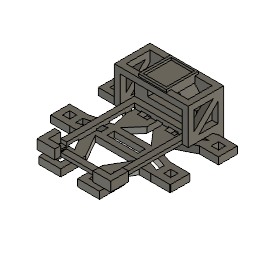
Proto-Board housing (Autodesk Fusion 360 design; units mm, degrees)
Autodesk Fusion 360 part; units mm, degrees
(part 1 of 2)
sketch "Sketch1" plane through (0, 0, 0) normal (0, 0, 1) x (1, 0, 0)
  line L0 (0, 0) -> (7, 0) construction
  line L1 (7, 0) -> (7, -7) construction
  line L2 (7, -7) -> (0, -7) construction
  line L3 (0, -7) -> (0, 0) construction
  line L4 (7, -3.5) -> (23, -3.5) construction
  line L5 (23, 0) -> (30, 0) construction
  line L6 (30, 0) -> (30, -7) construction
  line L7 (30, -7) -> (23, -7) construction
  line L8 (23, -7) -> (23, 0) construction
  line L9 (0, 0) -> (-25, 0) construction
  line L10 (30, 0) -> (55, 0) construction
  line L11 (-25, 0) -> (-30, 0) construction
  line L12 (-30, 0) -> (-30, 5) construction
  line L13 (-30, 5) -> (-25, 5) construction
  line L14 (-25, 5) -> (-25, 0) construction
  line L15 (55, 0) -> (60, 0) construction
  line L16 (60, 0) -> (60, 5) construction
  line L17 (60, 5) -> (55, 5) construction
  line L18 (55, 5) -> (55, 0) construction
  line L19 (-25, 0) -> (-25, -35) construction
  line L20 (-30, -35) -> (-25, -35) construction
  line L21 (-25, -35) -> (-25, -40) construction
  line L22 (-25, -40) -> (-30, -40) construction
  line L23 (-30, -40) -> (-30, -35) construction
  line L24 (55, 0) -> (55, -35) construction
  line L25 (55, -35) -> (60, -35) construction
  line L26 (60, -35) -> (60, -40) construction
  line L27 (60, -40) -> (55, -40) construction
  line L28 (55, -40) -> (55, -35) construction
  line L29 (15, -3.5) -> (15, -30) construction
  line L30 (15, -30) -> (2.5, -30) construction
  line L31 (2.5, -30) -> (27.5, -30) construction
  line L32 (27.5, -30) -> (27.5, -35) construction
  line L33 (27.5, -35) -> (2.5, -35) construction
  line L34 (2.5, -35) -> (2.5, -30) construction
  line L35 (2.5, -35) -> (2.5, -65) construction
  line L36 (27.5, -35) -> (27.5, -65) construction
  line L37 (2.5, -65) -> (-5, -65) construction
  line L38 (-5, -65) -> (-5, -75) construction
  line L39 (-5, -75) -> (2.5, -75) construction
  line L40 (2.5, -75) -> (2.5, -65) construction
  line L41 (27.5, -65) -> (35, -65) construction
  line L42 (35, -65) -> (35, -75) construction
  line L43 (35, -75) -> (27.5, -75) construction
  line L44 (27.5, -75) -> (27.5, -65) construction
  line L45 (-5, -65) -> (-5.5, -65) construction
  line L46 (-5.5, -65) -> (-5.5, -64.5) construction
  line L47 (-5.5, -64.5) -> (-5, -64.5) construction
  line L48 (-5, -64.5) -> (-5, -65) construction
  line L49 (-5.5, -64.5) -> (3, -64.5)
  line L50 (3, -64.5) -> (3, -75.5)
  line L51 (3, -75.5) -> (-5.5, -75.5)
  line L52 (-5.5, -75.5) -> (-5.5, -64.5)
  line L53 (27.5, -65) -> (27, -65) construction
  line L54 (27, -65) -> (27, -64.5) construction
  line L55 (27, -64.5) -> (27.5, -64.5) construction
  line L56 (27.5, -64.5) -> (27.5, -65) construction
  line L57 (27, -64.5) -> (35.5, -64.5)
  line L58 (35.5, -64.5) -> (35.5, -75.5)
  line L59 (35.5, -75.5) -> (27, -75.5)
  line L60 (27, -75.5) -> (27, -64.5)
  line L61 (2.5, -30) -> (2, -30) construction
  line L62 (2, -30) -> (2, -29.5) construction
  line L63 (2, -29.5) -> (2.5, -29.5) construction
  line L64 (2.5, -29.5) -> (2.5, -30) construction
  line L65 (-30, -35) -> (-30.5, -35) construction
  line L66 (-30.5, -35) -> (-30.5, -34.5) construction
  line L67 (-30.5, -34.5) -> (-30, -34.5) construction
  line L68 (-30, -34.5) -> (-30, -35) construction
  line L69 (-30.5, -34.5) -> (-24.5, -34.5)
  line L70 (-24.5, -34.5) -> (-24.5, -40.5)
  line L71 (-24.5, -40.5) -> (-30.5, -40.5)
  line L72 (-30.5, -40.5) -> (-30.5, -34.5)
  line L73 (-30, 5) -> (-30.5, 5) construction
  line L74 (-30.5, 5) -> (-30.5, 5.5) construction
  line L75 (-30.5, 5.5) -> (-30, 5.5) construction
  line L76 (-30, 5.5) -> (-30, 5) construction
  line L77 (-30.5, 5.5) -> (-24.5, 5.5)
  line L78 (-24.5, 5.5) -> (-24.5, -0.5)
  line L79 (-24.5, -0.5) -> (-30.5, -0.5)
  line L80 (-30.5, -0.5) -> (-30.5, 5.5)
  line L81 (0, 0) -> (-0.5, 0) construction
  line L82 (-0.5, 0) -> (-0.5, 0.5) construction
  line L83 (-0.5, 0.5) -> (0, 0.5) construction
  line L84 (0, 0.5) -> (0, 0) construction
  line L85 (-0.5, 0.5) -> (7.5, 0.5)
  line L86 (7.5, 0.5) -> (7.5, -7.5)
  line L87 (7.5, -7.5) -> (-0.5, -7.5)
  line L88 (-0.5, -7.5) -> (-0.5, 0.5)
  line L89 (23, 0) -> (22.5, 0) construction
  line L90 (22.5, 0) -> (22.5, 0.5) construction
  line L91 (22.5, 0.5) -> (23, 0.5) construction
  line L92 (23, 0.5) -> (23, 0) construction
  line L93 (22.5, 0.5) -> (30.5, 0.5)
  line L94 (30.5, 0.5) -> (30.5, -7.5)
  line L95 (30.5, -7.5) -> (22.5, -7.5)
  line L96 (22.5, -7.5) -> (22.5, 0.5)
  line L97 (55, 5) -> (54.5, 5) construction
  line L98 (54.5, 5) -> (54.5, 5.5) construction
  line L99 (54.5, 5.5) -> (55, 5.5) construction
  line L100 (55, 5.5) -> (55, 5) construction
  line L101 (54.5, 5.5) -> (60.5, 5.5)
  line L102 (60.5, 5.5) -> (60.5, -0.5)
  line L103 (60.5, -0.5) -> (54.5, -0.5)
  line L104 (54.5, -0.5) -> (54.5, 5.5)
  line L105 (54.5, -34.5) -> (60.5, -34.5)
  line L106 (60.5, -34.5) -> (60.5, -40.5)
  line L107 (60.5, -40.5) -> (54.5, -40.5)
  line L108 (54.5, -40.5) -> (54.5, -34.5)
  line L109 (60.5, -40.5) -> (65.5, -40.5) construction
  line L110 (65.5, -40.5) -> (65.5, -45.5) construction
  line L111 (65.5, -45.5) -> (60.5, -45.5) construction
  line L112 (60.5, -45.5) -> (60.5, -40.5) construction
  line L113 (35.5, -75.5) -> (40.5, -75.5) construction
  line L114 (40.5, -75.5) -> (40.5, -80.5) construction
  line L115 (40.5, -80.5) -> (35.5, -80.5) construction
  line L116 (35.5, -80.5) -> (35.5, -75.5) construction
  line L117 (40.5, -80.5) -> (65.5, -45.5)
  line L118 (60.5, -0.5) -> (65.5, -0.5) construction
  line L119 (65.5, -0.5) -> (65.5, -45.5)
  line L120 (-5.5, -75.5) -> (-10.5, -75.5) construction
  line L121 (-10.5, -75.5) -> (-10.5, -80.5) construction
  line L122 (-10.5, -80.5) -> (-5.5, -80.5) construction
  line L123 (-5.5, -80.5) -> (-5.5, -75.5) construction
  line L124 (-10.5, -80.5) -> (40.5, -80.5)
  line L125 (-30.5, -40.5) -> (-35.5, -40.5) construction
  line L126 (-35.5, -40.5) -> (-35.5, -45.5) construction
  line L127 (-35.5, -45.5) -> (-30.5, -45.5) construction
  line L128 (-30.5, -45.5) -> (-30.5, -40.5) construction
  line L129 (-35.5, -45.5) -> (-10.5, -80.5)
  line L130 (2, -29.5) -> (28, -29.5)
  line L131 (28, -29.5) -> (28, -35.5)
  line L132 (28, -35.5) -> (2, -35.5)
  line L133 (2, -35.5) -> (2, -29.5)
  line L134 (-30.5, -0.5) -> (-35.5, -0.5) construction
  line L135 (-35.5, -45.5) -> (-35.5, -0.5)
  line L136 (-30.5, 5.5) -> (-35.5, 5.5) construction
  line L137 (-35.5, 5.5) -> (-35.5, 10.5) construction
  line L138 (-35.5, 10.5) -> (-30.5, 10.5) construction
  line L139 (-30.5, 10.5) -> (-30.5, 5.5) construction
  line L140 (-35.5, -0.5) -> (-35.5, 10.5)
  line L141 (-24.5, 5.5) -> (-19.5, 5.5) construction
  line L142 (-19.5, 5.5) -> (-19.5, 10.5) construction
  line L143 (-19.5, 10.5) -> (-24.5, 10.5) construction
  line L144 (-24.5, 10.5) -> (-24.5, 5.5) construction
  line L145 (-35.5, 10.5) -> (-19.5, 10.5)
  line L146 (-0.5, 0.5) -> (-5.5, 0.5) construction
  line L147 (-5.5, 0.5) -> (-5.5, 5.5) construction
  line L148 (-5.5, 5.5) -> (-0.5, 5.5) construction
  line L149 (-0.5, 5.5) -> (-0.5, 0.5) construction
  line L150 (-19.5, 10.5) -> (-5.5, 5.5)
  line L151 (7.5, 0.5) -> (12.5, 0.5) construction
  line L152 (12.5, 0.5) -> (12.5, 5.5) construction
  line L153 (12.5, 5.5) -> (7.5, 5.5) construction
  line L154 (7.5, 5.5) -> (7.5, 0.5) construction
  line L155 (-5.5, 5.5) -> (12.5, 5.5)
  line L156 (30.5, 0.5) -> (35.5, 0.5) construction
  line L157 (35.5, 0.5) -> (35.5, 5.5) construction
  line L158 (35.5, 5.5) -> (30.5, 5.5) construction
  line L159 (30.5, 5.5) -> (30.5, 0.5) construction
  line L160 (12.5, 5.5) -> (35.5, 5.5)
  line L161 (54.5, 5.5) -> (49.5, 5.5) construction
  line L162 (49.5, 5.5) -> (49.5, 10.5) construction
  line L163 (49.5, 10.5) -> (54.5, 10.5) construction
  line L164 (54.5, 10.5) -> (54.5, 5.5) construction
  line L165 (35.5, 5.5) -> (49.5, 10.5)
  line L166 (60.5, 5.5) -> (65.5, 5.5) construction
  line L167 (65.5, 5.5) -> (65.5, 10.5) construction
  line L168 (65.5, 10.5) -> (60.5, 10.5) construction
  line L169 (60.5, 10.5) -> (60.5, 5.5) construction
  line L170 (49.5, 10.5) -> (65.5, 10.5)
  line L171 (65.5, 10.5) -> (65.5, -0.5)
  line L172 (30.5, -7.5) -> (35.5, -7.5) construction
  line L173 (35.5, -7.5) -> (35.5, -12.5) construction
  line L174 (35.5, -12.5) -> (30.5, -12.5) construction
  line L175 (30.5, -12.5) -> (30.5, -7.5) construction
  line L176 (54.5, -0.5) -> (49.5, -0.5) construction
  line L177 (49.5, -0.5) -> (49.5, -5.5) construction
  line L178 (49.5, -5.5) -> (54.5, -5.5) construction
  line L179 (54.5, -5.5) -> (54.5, -0.5) construction
  line L180 (54.5, -34.5) -> (49.5, -34.5) construction
  line L181 (49.5, -34.5) -> (49.5, -29.5) construction
  line L182 (49.5, -29.5) -> (54.5, -29.5) construction
  line L183 (54.5, -29.5) -> (54.5, -34.5) construction
  line L184 (28, -29.5) -> (33, -29.5) construction
  line L185 (33, -29.5) -> (33, -24.5) construction
  line L186 (33, -24.5) -> (28, -24.5) construction
  line L187 (28, -24.5) -> (28, -29.5) construction
  line L188 (33, -24.5) -> (35.5, -12.5)
  line L189 (35.5, -12.5) -> (49.5, -5.5)
  line L190 (49.5, -5.5) -> (49.5, -29.5)
  line L191 (33, -24.5) -> (49.5, -29.5)
  line L192 (7.5, -7.5) -> (12.5, -7.5) construction
  line L193 (12.5, -7.5) -> (12.5, -12.5) construction
  line L194 (12.5, -12.5) -> (7.5, -12.5) construction
  line L195 (7.5, -12.5) -> (7.5, -7.5) construction
  line L196 (22.5, -7.5) -> (17.5, -7.5) construction
  line L197 (17.5, -7.5) -> (17.5, -12.5) construction
  line L198 (17.5, -12.5) -> (22.5, -12.5) construction
  line L199 (22.5, -12.5) -> (22.5, -7.5) construction
  line L200 (-0.5, -7.5) -> (-5.5, -7.5) construction
  line L201 (-5.5, -7.5) -> (-5.5, -12.5) construction
  line L202 (-5.5, -12.5) -> (-0.5, -12.5) construction
  line L203 (-0.5, -12.5) -> (-0.5, -7.5) construction
  line L204 (2, -29.5) -> (-3, -29.5) construction
  line L205 (-3, -29.5) -> (-3, -24.5) construction
  line L206 (-3, -24.5) -> (2, -24.5) construction
  line L207 (2, -24.5) -> (2, -29.5) construction
  line L208 (-24.5, -0.5) -> (-19.5, -0.5) construction
  line L209 (-19.5, -0.5) -> (-19.5, -5.5) construction
  line L210 (-19.5, -5.5) -> (-24.5, -5.5) construction
  line L211 (-24.5, -5.5) -> (-24.5, -0.5) construction
  line L212 (-24.5, -34.5) -> (-19.5, -34.5) construction
  line L213 (-19.5, -34.5) -> (-19.5, -29.5) construction
  line L214 (-19.5, -29.5) -> (-24.5, -29.5) construction
  line L215 (-24.5, -29.5) -> (-24.5, -34.5) construction
  line L216 (-19.5, -5.5) -> (-19.5, -29.5)
  line L217 (-19.5, -29.5) -> (-3, -24.5)
  line L218 (-3, -24.5) -> (-5.5, -12.5)
  line L219 (-5.5, -12.5) -> (-19.5, -5.5)
  line L220 (3, -64.5) -> (8, -64.5) construction
  line L221 (8, -64.5) -> (8, -59.5) construction
  line L222 (8, -59.5) -> (3, -59.5) construction
  line L223 (3, -59.5) -> (3, -64.5) construction
  line L224 (27, -64.5) -> (22, -64.5) construction
  line L225 (22, -64.5) -> (22, -59.5) construction
  line L226 (22, -59.5) -> (27, -59.5) construction
  line L227 (27, -59.5) -> (27, -64.5) construction
  line L228 (2, -35.5) -> (-3, -35.5) construction
  line L229 (-3, -35.5) -> (-3, -40.5) construction
  line L230 (-3, -40.5) -> (2, -40.5) construction
  line L231 (2, -40.5) -> (2, -35.5) construction
  line L232 (28, -35.5) -> (33, -35.5) construction
  line L233 (33, -35.5) -> (33, -40.5) construction
  line L234 (33, -40.5) -> (28, -40.5) construction
  line L235 (28, -40.5) -> (28, -35.5) construction
  line L236 (-3, -40.5) -> (8, -59.5)
  line L237 (8, -59.5) -> (22, -59.5)
  line L238 (22, -59.5) -> (33, -40.5)
  line L239 (33, -40.5) -> (-3, -40.5)
  dimension "d1" = 7
  dimension "d2" = 7
  dimension "d3" = 16
  dimension "d4" = 25
  dimension "d5" = 25
  dimension "d6" = 26.5
  dimension "d7" = 12.5
  dimension "d8" = 25
  dimension "d9" = 5
  dimension "d10" = 30
  dimension "d11" = 7.5
  dimension "d12" = 10
  dimension "d13" = 7.5
  dimension "d14" = 10
  dimension "d15" = 0.5
  dimension "d16" = 0.5
  dimension "d17" = 8.5
  dimension "d18" = 11
  dimension "d19" = 0.5
  dimension "d20" = 0.5
  dimension "d21" = 8.5
  dimension "d22" = 11
  dimension "d23" = 0.5
  dimension "d24" = 0.5
  dimension "d27" = 5
  dimension "d28" = 5
  dimension "d29" = 5
  dimension "d30" = 5
  dimension "d31" = 5
  dimension "d32" = 5
  dimension "d33" = 5
  dimension "d34" = 5
  dimension "d35" = 5
  dimension "d36" = 26
  dimension "d37" = 6
  dimension "d38" = 5
  dimension "d39" = 5
  dimension "d40" = 5
  dimension "d41" = 5
  dimension "d42" = 5
  dimension "d43" = 5
  dimension "d44" = 5
  dimension "d45" = 5
  dimension "d46" = 5
  dimension "d47" = 5
  dimension "d48" = 5
  dimension "d49" = 5
  dimension "d50" = 5
  dimension "d51" = 5
  dimension "d52" = 5
  dimension "d53" = 5
  dimension "d54" = 5
  dimension "d55" = 5
  dimension "d56" = 5
  dimension "d57" = 5
  dimension "d58" = 5
  dimension "d59" = 5
  dimension "d60" = 5
  dimension "d61" = 5
  dimension "d62" = 5
  dimension "d63" = 5
  dimension "d64" = 5
  dimension "d65" = 5
  dimension "d66" = 5
  dimension "d67" = 5
  dimension "d68" = 5
  dimension "d69" = 5
  dimension "d70" = 5
  dimension "d71" = 5
  dimension "d72" = 5
  dimension "d73" = 5
  dimension "d74" = 5
  dimension "d75" = 5
  dimension "d76" = 5
  dimension "d77" = 5
  dimension "d78" = 5
  dimension "d79" = 5
  dimension "d80" = 5
  constraint horizontal L0
  constraint vertical L1
  constraint horizontal L2
  constraint vertical L3
  constraint coincident L0.start L3.end
  constraint midpoint L1 L4.start
  constraint perpendicular L1 L4
  constraint horizontal L5
  constraint vertical L6
  constraint horizontal L7
  constraint vertical L8
  constraint perpendicular L3 L9
  constraint perpendicular L6 L10
  constraint horizontal L11
  constraint vertical L12
  constraint horizontal L13
  constraint vertical L14
  constraint horizontal L15
  constraint vertical L16
  constraint horizontal L17
  constraint vertical L18
  constraint perpendicular L11 L19
  constraint horizontal L20
  constraint vertical L21
  constraint horizontal L22
  constraint vertical L23
  constraint perpendicular L10 L24
  constraint horizontal L25
  constraint vertical L26
  constraint horizontal L27
  constraint vertical L28
  constraint midpoint L4 L29.start
  constraint perpendicular L4 L29
  constraint perpendicular L29 L30
  constraint horizontal L31
  constraint vertical L32
  constraint horizontal L33
  constraint vertical L34
  constraint perpendicular L33 L35
  constraint perpendicular L33 L36
  constraint horizontal L37
  constraint vertical L38
  constraint horizontal L39
  constraint vertical L40
  constraint horizontal L41
  constraint vertical L42
  constraint horizontal L43
  constraint vertical L44
  constraint horizontal L45
  constraint vertical L46
  constraint horizontal L47
  constraint vertical L48
  constraint horizontal L49
  constraint vertical L50
  constraint horizontal L51
  constraint vertical L52
  constraint horizontal L53
  constraint vertical L54
  constraint horizontal L55
  constraint vertical L56
  constraint horizontal L57
  constraint vertical L58
  constraint horizontal L59
  constraint vertical L60
  constraint horizontal L61
  constraint vertical L62
  constraint horizontal L63
  constraint vertical L64
  constraint horizontal L65
  constraint vertical L66
  constraint horizontal L67
  constraint vertical L68
  constraint horizontal L69
  constraint vertical L70
  constraint horizontal L71
  constraint vertical L72
  constraint horizontal L73
  constraint vertical L74
  constraint horizontal L75
  constraint vertical L76
  constraint horizontal L77
  constraint vertical L78
  constraint horizontal L79
  constraint vertical L80
  constraint horizontal L81
  constraint vertical L82
  constraint horizontal L83
  constraint vertical L84
  constraint horizontal L85
  constraint vertical L86
  constraint horizontal L87
  constraint vertical L88
  constraint horizontal L89
  constraint vertical L90
  constraint horizontal L91
  constraint vertical L92
  constraint horizontal L93
  constraint vertical L94
  constraint horizontal L95
  constraint vertical L96
  constraint horizontal L97
  constraint vertical L98
  constraint horizontal L99
  constraint vertical L100
  constraint horizontal L101
  constraint vertical L102
  constraint horizontal L103
  constraint vertical L104
  constraint horizontal L105
  constraint vertical L106
  constraint horizontal L107
  constraint vertical L108
  constraint horizontal L109
  constraint vertical L110
  constraint horizontal L111
  constraint vertical L112
  constraint horizontal L113
  constraint vertical L114
  constraint horizontal L115
  constraint vertical L116
  constraint perpendicular L102 L118
  constraint perpendicular L111 L119
  constraint horizontal L120
  constraint vertical L121
  constraint horizontal L122
  constraint vertical L123
  constraint horizontal L125
  constraint vertical L126
  constraint horizontal L127
  constraint vertical L128
  constraint horizontal L130
  constraint vertical L131
  constraint horizontal L132
  constraint vertical L133
  constraint perpendicular L80 L134
  constraint perpendicular L134 L135
  constraint horizontal L136
  constraint vertical L137
  constraint horizontal L138
  constraint vertical L139
  constraint horizontal L141
  constraint vertical L142
  constraint horizontal L143
  constraint vertical L144
  constraint horizontal L146
  constraint vertical L147
  constraint horizontal L148
  constraint vertical L149
  constraint horizontal L151
  constraint vertical L152
  constraint horizontal L153
  constraint vertical L154
  constraint horizontal L156
  constraint vertical L157
  constraint horizontal L158
  constraint vertical L159
  constraint perpendicular L157 L160
  constraint horizontal L161
  constraint vertical L162
  constraint horizontal L163
  constraint vertical L164
  constraint horizontal L166
  constraint vertical L167
  constraint horizontal L168
  constraint vertical L169
  constraint horizontal L172
  constraint vertical L173
  constraint horizontal L174
  constraint vertical L175
  constraint horizontal L176
  constraint vertical L177
  constraint horizontal L178
  constraint vertical L179
  constraint horizontal L180
  constraint vertical L181
  constraint horizontal L182
  constraint vertical L183
  constraint horizontal L184
  constraint vertical L185
  constraint horizontal L186
  constraint vertical L187
  constraint perpendicular L182 L190
  constraint horizontal L192
  constraint vertical L193
  constraint horizontal L194
  constraint vertical L195
  constraint horizontal L196
  constraint vertical L197
  constraint horizontal L198
  constraint vertical L199
  constraint horizontal L200
  constraint vertical L201
  constraint horizontal L202
  constraint vertical L203
  constraint horizontal L204
  constraint vertical L205
  constraint horizontal L206
  constraint vertical L207
  constraint horizontal L208
  constraint vertical L209
  constraint horizontal L210
  constraint vertical L211
  constraint horizontal L212
  constraint vertical L213
  constraint horizontal L214
  constraint vertical L215
  constraint perpendicular L214 L216
  constraint horizontal L220
  constraint vertical L221
  constraint horizontal L222
  constraint vertical L223
  constraint horizontal L224
  constraint vertical L225
  constraint horizontal L226
  constraint vertical L227
  constraint horizontal L228
  constraint vertical L229
  constraint horizontal L230
  constraint vertical L231
  constraint horizontal L232
  constraint vertical L233
  constraint horizontal L234
  constraint vertical L235
  measures "d1" distance of L0.start L0.end
  measures "d2" distance of L0.start L2.end
  measures "d3" distance of L4.start L4.end
  measures "d4" distance of L0.start L9.end
  measures "d5" distance of L5.end L10.end
  measures "d6" distance of L29.start L29.end
  measures "d7" distance of L29.end L30.end
  measures "d8" distance of L30.end L31.end
  measures "d9" distance of L30.end L33.end
  measures "d10" distance of L33.end L35.end
  measures "d11" distance of L35.end L37.end
  measures "d12" distance of L35.end L39.end
  measures "d13" distance of L36.end L41.end
  measures "d14" distance of L36.end L43.end
  measures "d15" distance of L37.end L45.end
  measures "d16" distance of L37.end L47.end
  measures "d17" distance of L46.end L49.end
  measures "d18" distance of L46.end L51.end
  measures "d19" distance of L36.end L53.end
  measures "d20" distance of L36.end L55.end
  measures "d21" distance of L54.end L57.end
  measures "d22" distance of L54.end L59.end
  measures "d23" distance of L30.end L61.end
  measures "d24" distance of L30.end L63.end
  measures "d27" distance of L106.end L109.end
  measures "d28" distance of L106.end L111.end
  measures "d29" distance of L58.end L113.end
  measures "d30" distance of L58.end L115.end
  measures "d31" distance of L102.end L118.end
  measures "d32" distance of L51.end L120.end
  measures "d33" distance of L51.end L122.end
  measures "d34" distance of L71.end L125.end
  measures "d35" distance of L71.end L127.end
  measures "d36" distance of L62.end L130.end
  measures "d37" distance of L62.end L132.end
  measures "d38" distance of L79.end L134.end
  measures "d39" distance of L74.end L136.end
  measures "d40" distance of L74.end L138.end
  measures "d41" distance of L77.end L141.end
  measures "d42" distance of L77.end L143.end
  measures "d43" distance of L82.end L146.end
  measures "d44" distance of L82.end L148.end
  measures "d45" distance of L85.end L151.end
  measures "d46" distance of L85.end L153.end
  measures "d47" distance of L93.end L156.end
  measures "d48" distance of L93.end L158.end
  measures "d49" distance of L98.end L161.end
  measures "d50" distance of L98.end L163.end
  measures "d51" distance of L101.end L166.end
  measures "d52" distance of L101.end L168.end
  measures "d53" distance of L94.end L172.end
  measures "d54" distance of L94.end L174.end
  measures "d55" distance of L103.end L176.end
  measures "d56" distance of L103.end L178.end
  measures "d57" distance of L105.start L180.end
  measures "d58" distance of L105.start L182.end
  measures "d59" distance of L130.end L184.end
  measures "d60" distance of L130.end L186.end
  measures "d61" distance of L86.end L192.end
  measures "d62" distance of L86.end L194.end
  measures "d63" distance of L95.end L196.end
  measures "d64" distance of L95.end L198.end
  measures "d65" distance of L87.end L200.end
  measures "d66" distance of L87.end L202.end
  measures "d67" distance of L62.end L204.end
  measures "d68" distance of L62.end L206.end
  measures "d69" distance of L78.end L208.end
  measures "d70" distance of L78.end L210.end
  measures "d71" distance of L69.end L212.end
  measures "d72" distance of L69.end L214.end
  measures "d73" distance of L49.end L220.end
  measures "d74" distance of L49.end L222.end
  measures "d75" distance of L54.end L224.end
  measures "d76" distance of L54.end L226.end
  measures "d77" distance of L132.end L228.end
  measures "d78" distance of L132.end L230.end
  measures "d79" distance of L131.end L232.end
  measures "d80" distance of L131.end L234.end
extrude "Extrude1" add sketch "Sketch1" along normal blind 6
sketch "Sketch2" plane through (0, 5.5, 0) normal (0, 1, 0) x (-1, 0, 0)
  line L0 (-35.5, 0) -> (5.5, 0)
  line L1 (5.5, 0) -> (5.5, 6)
  line L2 (5.5, 6) -> (-35.5, 6)
  line L3 (-35.5, 6) -> (-35.5, 0)
  line L4 (-15, 6) -> (-15, 0) construction
  line L5 (-15, 3) -> (-38, 3) construction
  line L6 (-38, 3) -> (-39, 3) construction
  line L7 (-39, 3) -> (-39, 6) construction
  line L8 (-39, 6) -> (-44, 6) construction
  line L9 (-44, 6) -> (-44, -9) construction
  line L10 (-44, -9) -> (14, -9)
  line L11 (14, -9) -> (14, 21)
  line L12 (14, 21) -> (-44, 21)
  line L13 (-44, 21) -> (-44, -9)
  line L14 (-44, 21) -> (-39, 21) construction
  line L15 (-39, 21) -> (-39, 16) construction
  line L16 (-39, 16) -> (-44, 16) construction
  line L17 (-44, 16) -> (-44, 21) construction
  line L18 (-39, 17) -> (9, 17)
  line L19 (9, 17) -> (9, -5)
  line L20 (9, -5) -> (-39, -5)
  line L21 (-39, -5) -> (-39, 17)
  dimension "d83" = 5
  dimension "d84" = 58
  dimension "d85" = 30
  dimension "d86" = 5
  dimension "d87" = 5
  dimension "d88" = 48
  dimension "d89" = 22
  constraint midpoint L2 L4.start
  constraint midpoint L0 L4.end
  constraint midpoint L4 L5.start
  constraint perpendicular L3 L5
  constraint perpendicular L3 L6
  constraint perpendicular L6 L7
  constraint perpendicular L7 L8
  constraint perpendicular L8 L9
  constraint horizontal L10
  constraint vertical L11
  constraint horizontal L12
  constraint vertical L13
  constraint horizontal L14
  constraint vertical L15
  constraint horizontal L16
  constraint vertical L17
  constraint horizontal L18
  constraint vertical L19
  constraint horizontal L20
  constraint vertical L21
  constraint coincident L15 L18.start
  measures "d83" distance of L7.end L8.end
  measures "d84" distance of L9.end L10.end
  measures "d85" distance of L9.end L12.end
  measures "d86" distance of L12.end L14.end
  measures "d87" distance of L12.end L16.end
  measures "d88" distance of L18.start L18.end
  measures "d89" distance of L18.start L20.end
extrude "Extrude2" add sketch "Sketch2" along normal blind 13 contours L0 L1 L2 L3 | L10 L11 L12 L13 | L18 L19 L20 L21
sketch "Sketch3" plane through (0, 18.5, 0) normal (0, 1, 0) x (-1, 0, 0)
  line L0 (-44, 21) -> (-44, -9)
  line L1 (-44, -9) -> (14, -9)
  line L2 (14, -9) -> (14, 21)
  line L3 (14, 21) -> (-44, 21)
  line L4 (-44, 21) -> (-40, 21) construction
  line L5 (-40, 21) -> (-40, 17) construction
  line L6 (-40, 17) -> (-44, 17) construction
  line L7 (-44, 17) -> (-44, 21) construction
  line L8 (-40, 17) -> (10, 17)
  line L9 (10, 17) -> (10, -5)
  line L10 (10, -5) -> (-40, -5)
  line L11 (-40, -5) -> (-40, 17)
  dimension "d92" = 4
  dimension "d93" = 4
  dimension "d94" = 50
  dimension "d95" = 22
  constraint horizontal L4
  constraint vertical L5
  constraint horizontal L6
  constraint vertical L7
  constraint coincident L0.start L3.end
  constraint horizontal L8
  constraint vertical L9
  constraint horizontal L10
  constraint vertical L11
  measures "d92" distance of L0.start L4.end
  measures "d93" distance of L0.start L6.end
  measures "d94" distance of L5.end L8.end
  measures "d95" distance of L5.end L10.end
extrude "Extrude3" cut sketch "Sketch3" against normal blind 10 contours L8 L9 L10 L11
sketch "Sketch4" plane through (0, 18.5, 0) normal (0, 1, 0) x (-1, 0, 0)
  line L0 (10, 17) -> (10, -5)
  line L1 (10, -5) -> (-40, -5)
  line L2 (-40, -5) -> (-40, 17)
  line L3 (-40, 17) -> (10, 17)
  line L4 (-44, 21) -> (-44, -9)
  line L5 (-44, -9) -> (14, -9)
  line L6 (14, -9) -> (14, 21)
  line L7 (14, 21) -> (-44, 21)
  line L8 (-15, 17) -> (-15, 21) construction
  line L9 (-15, 21) -> (-30, 21) construction
  line L10 (-30, 21) -> (0, 21)
  line L11 (0, 21) -> (0, 17)
  line L12 (0, 17) -> (-30, 17)
  line L13 (-30, 17) -> (-30, 21)
  dimension "d98" = 15
  dimension "d99" = 30
  constraint midpoint L3 L8.start
  constraint midpoint L7 L8.end
  constraint perpendicular L8 L9
  constraint horizontal L10
  constraint vertical L11
  constraint horizontal L12
  constraint vertical L13
  measures "d98" distance of L8.end L9.end
  measures "d99" distance of L9.end L10.end
extrude "Extrude4" cut sketch "Sketch4" against normal blind 10 contours L3 L7 L10 L11 L12 L13
sketch "Sketch5" plane through (0, 0, 6) normal (0, 0, 1) x (-1, 0, 0)
  line L0 (14, -5.5) -> (14, -8.5357)
  line L1 (14, -8.5357) -> (19.5, -10.5)
  line L2 (19.5, -10.5) -> (35.5, -10.5)
  line L3 (35.5, -10.5) -> (35.5, 45.5)
  line L4 (35.5, 45.5) -> (10.5, 80.5)
  line L5 (10.5, 80.5) -> (-40.5, 80.5)
  line L6 (-40.5, 80.5) -> (-65.5, 45.5)
  line L7 (-65.5, 45.5) -> (-65.5, -10.5)
  line L8 (-65.5, -10.5) -> (-49.5, -10.5)
  line L9 (-49.5, -10.5) -> (-44, -8.5357)
  line L10 (-44, -8.5357) -> (-44, -5.5)
  line L11 (-44, -5.5) -> (14, -5.5)
  line L12 (19.5, 5.5) -> (5.5, 12.5)
  line L13 (5.5, 12.5) -> (3, 24.5)
  line L14 (3, 24.5) -> (19.5, 29.5)
  line L15 (19.5, 29.5) -> (19.5, 5.5)
  line L16 (3, 40.5) -> (-33, 40.5)
  line L17 (-33, 40.5) -> (-22, 59.5)
  line L18 (-22, 59.5) -> (-8, 59.5)
  line L19 (-8, 59.5) -> (3, 40.5)
  line L20 (-3, 75.5) -> (5.5, 75.5)
  line L21 (5.5, 75.5) -> (5.5, 64.5)
  line L22 (5.5, 64.5) -> (-3, 64.5)
  line L23 (-3, 64.5) -> (-3, 75.5)
  line L24 (-30.5, 7.5) -> (-22.5, 7.5)
  line L25 (-22.5, 7.5) -> (-22.5, -0.5)
  line L26 (-22.5, -0.5) -> (-30.5, -0.5)
  line L27 (-30.5, -0.5) -> (-30.5, 7.5)
  line L28 (24.5, 40.5) -> (30.5, 40.5)
  line L29 (30.5, 40.5) -> (30.5, 34.5)
  line L30 (30.5, 34.5) -> (24.5, 34.5)
  line L31 (24.5, 34.5) -> (24.5, 40.5)
  line L32 (-28, 35.5) -> (-2, 35.5)
  line L33 (-2, 35.5) -> (-2, 29.5)
  line L34 (-2, 29.5) -> (-28, 29.5)
  line L35 (-28, 29.5) -> (-28, 35.5)
  line L36 (-7.5, 7.5) -> (0.5, 7.5)
  line L37 (0.5, 7.5) -> (0.5, -0.5)
  line L38 (0.5, -0.5) -> (-7.5, -0.5)
  line L39 (-7.5, -0.5) -> (-7.5, 7.5)
  line L40 (24.5, 0.5) -> (30.5, 0.5)
  line L41 (30.5, 0.5) -> (30.5, -5.5)
  line L42 (30.5, -5.5) -> (24.5, -5.5)
  line L43 (24.5, -5.5) -> (24.5, 0.5)
  line L44 (-60.5, 40.5) -> (-54.5, 40.5)
  line L45 (-54.5, 40.5) -> (-54.5, 34.5)
  line L46 (-54.5, 34.5) -> (-60.5, 34.5)
  line L47 (-60.5, 34.5) -> (-60.5, 40.5)
  line L48 (-60.5, 0.5) -> (-54.5, 0.5)
  line L49 (-54.5, 0.5) -> (-54.5, -5.5)
  line L50 (-54.5, -5.5) -> (-60.5, -5.5)
  line L51 (-60.5, -5.5) -> (-60.5, 0.5)
  line L52 (-35.5, 75.5) -> (-27, 75.5)
  line L53 (-27, 75.5) -> (-27, 64.5)
  line L54 (-27, 64.5) -> (-35.5, 64.5)
  line L55 (-35.5, 64.5) -> (-35.5, 75.5)
  line L56 (-33, 24.5) -> (-35.5, 12.5)
  line L57 (-35.5, 12.5) -> (-49.5, 5.5)
  line L58 (-49.5, 5.5) -> (-49.5, 29.5)
  line L59 (-49.5, 29.5) -> (-33, 24.5)
  line L60 (-15, -5.5) -> (-15, 76.5) construction
  line L61 (-15, 76.5) -> (16, 76.5) construction
  line L62 (16, 76.5) -> (-46, 76.5)
  line L63 (-46, 76.5) -> (-46, -5.5)
  line L64 (-46, -5.5) -> (16, -5.5)
  line L65 (16, -5.5) -> (16, 76.5)
  dimension "d102" = 82
  dimension "d103" = 31
  dimension "d104" = 62
  constraint midpoint L11 L60.start
  constraint perpendicular L5 L60
  constraint perpendicular L21 L61
  constraint horizontal L62
  constraint vertical L63
  constraint horizontal L64
  constraint vertical L65
  measures "d102" distance of L60.start L60.end
  measures "d103" distance of L60.end L61.end
  measures "d104" distance of L61.end L62.end
extrude "Extrude5" add sketch "Sketch5" along normal blind 3 contours L4 L6 L11 L12 L13 L14 L56 L57 L59 L62 L63 L64 L65 | L12 L13 L14 L65 | L56 L57 L59 L63 | L4 L62 L65 | L6 L62 L63 | L16 L17 L18 L19 | L20 L21 L22 L23 | L24 L25 L26 L27 | L32 L33 L34 L35 | L36 L37 L38 L39 | L52 L53 L54 L55
sketch "Sketch6" plane through (0, 0, 9) normal (0, 0, 1) x (-1, 0, 0)
  line L0 (16, -5.5) -> (16, 76.5)
  line L1 (16, 76.5) -> (-46, 76.5)
  line L2 (-46, 76.5) -> (-46, -5.5)
  line L3 (-46, -5.5) -> (-44, -5.5)
  line L4 (-44, -5.5) -> (14, -5.5)
  line L5 (14, -5.5) -> (16, -5.5)
  line L6 (16, -5.5) -> (11, -5.5) construction
  line L7 (11, -5.5) -> (11, -0.5) construction
  line L8 (11, -0.5) -> (16, -0.5) construction
  line L9 (16, -0.5) -> (16, -5.5) construction
  line L10 (11, -0.5) -> (-41, -0.5)
  line L11 (-41, -0.5) -> (-41, 71.5)
  line L12 (-41, 71.5) -> (11, 71.5)
  line L13 (11, 71.5) -> (11, -0.5)
  dimension "d107" = 5
  dimension "d108" = 5
  dimension "d109" = 52
  dimension "d110" = 72
  constraint horizontal L6
  constraint vertical L7
  constraint horizontal L8
  constraint vertical L9
  constraint coincident L0.start L5.end
  constraint horizontal L10
  constraint vertical L11
  constraint horizontal L12
  constraint vertical L13
  measures "d107" distance of L0.start L6.end
  measures "d108" distance of L0.start L8.end
  measures "d109" distance of L7.end L10.end
  measures "d110" distance of L7.end L12.end
extrude "Extrude6" add sketch "Sketch6" along normal blind 5
sketch "Sketch7" plane through (0, 0, 9) normal (0, 0, 1) x (-1, 0, 0)
  line L0 (-41, 71.5) -> (-41, -0.5)
  line L1 (-41, -0.5) -> (11, -0.5)
  line L2 (11, -0.5) -> (11, 71.5)
  line L3 (11, 71.5) -> (-41, 71.5)
  line L4 (11, -0.5) -> (6, -0.5) construction
  line L5 (6, -0.5) -> (6, 4.5) construction
  line L6 (6, 4.5) -> (11, 4.5) construction
  line L7 (11, 4.5) -> (11, -0.5) construction
  line L8 (6, 4.5) -> (-36, 4.5)
  line L9 (-36, 4.5) -> (-36, 66.5)
  line L10 (-36, 66.5) -> (6, 66.5)
  line L11 (6, 66.5) -> (6, 4.5)
  dimension "d113" = 5
  dimension "d114" = 5
  dimension "d115" = 42
  dimension "d116" = 62
  constraint horizontal L4
  constraint vertical L5
  constraint horizontal L6
  constraint vertical L7
  constraint coincident L1.end L2.start
  constraint horizontal L8
  constraint vertical L9
  constraint horizontal L10
  constraint vertical L11
  measures "d113" distance of L1.end L4.end
  measures "d114" distance of L1.end L6.end
  measures "d115" distance of L5.end L8.end
  measures "d116" distance of L5.end L10.end
extrude "Extrude7" cut sketch "Sketch7" against normal blind 4 contours L8 L9 L10 L11
sketch "Sketch8" plane through (30, 0, 0) normal (-1, 0, 0) x (0, -1, 0)
  line L0 (-18.5, 21) -> (-18.5, 17)
  line L1 (-18.5, 17) -> (-8.5, 17)
  line L2 (-8.5, 17) -> (-8.5, 21)
  line L3 (-8.5, 21) -> (-18.5, 21)
  line L4 (-18.5, 21) -> (-14.5, 21)
  line L5 (-14.5, 21) -> (-14.5, 17)
  line L6 (-14.5, 17) -> (-18.5, 17)
  line L7 (-18.5, 17) -> (-18.5, 21)
  dimension "d119" = 4
  constraint horizontal L4
  constraint vertical L5
  constraint horizontal L6
  constraint vertical L7
  constraint coincident L0.start L3.end
  measures "d119" distance of L0.start L4.end
extrude "Extrude8" add sketch "Sketch8" along normal blind 30 contours L0 L1 L3 L4 L5 L6 L7
sketch "Sketch9" plane through (0, 0, 21) normal (0, 0, 1) x (-1, 0, 0)
  line L0 (-44, -18.5) -> (14, -18.5)
  line L1 (14, -18.5) -> (14, -5.5)
  line L2 (14, -5.5) -> (-44, -5.5)
  line L3 (-44, -5.5) -> (-44, -18.5)
  line L4 (0, -14.5) -> (-30, -14.5)
  line L5 (-30, -14.5) -> (-30, -8.5)
  line L6 (-30, -8.5) -> (0, -8.5)
  line L7 (0, -8.5) -> (0, -14.5)
  line L8 (-30, -8.5) -> (0, -8.5)
  line L9 (0, -8.5) -> (0, -5.5)
  line L10 (0, -5.5) -> (-30, -5.5)
  line L11 (-30, -5.5) -> (-30, -8.5)
  dimension "d122" = 30
  constraint horizontal L8
  constraint vertical L9
  constraint horizontal L10
  constraint vertical L11
  constraint coincident L5.end L6.start
  measures "d122" distance of L5.end L6.end
extrude "Extrude9" add sketch "Sketch9" along normal blind 10 contours L0 L1 L2 L3 L4 L5 L7 L9 L11
extrude "Extrude10" add 1 faces at (-14, 15.1786, 9.3333) along direction (-1, 0, 0) blind 2
extrude "Extrude11" add 1 faces at (44, 15.1786, 9.3333) along direction (1, 0, 0) blind 2
extrude "Extrude12" add 1 faces at (40.6667, 12.8333, 31) along direction (0, 0, 1) blind 5
sketch "Sketch10" plane through (0, 0, 0) normal (1, 0, 0) x (0, 1, 0)
  line L0 (14.5, 17) -> (14.5, 36)
  line L1 (14.5, 36) -> (5.5, 36)
  line L2 (5.5, 36) -> (5.5, 21)
  line L3 (5.5, 21) -> (8.5, 21)
  line L4 (8.5, 21) -> (8.5, 17)
  line L5 (8.5, 17) -> (14.5, 17)
  line L6 (5.5, 36) -> (14.5, 36)
  line L7 (14.5, 36) -> (14.5, 31)
  line L8 (14.5, 31) -> (5.5, 31)
  line L9 (5.5, 31) -> (5.5, 36)
  dimension "d131" = 5
  constraint horizontal L6
  constraint vertical L7
  constraint horizontal L8
  constraint vertical L9
  constraint coincident L1.end L2.start
  measures "d131" distance of L1.end L8.end
extrude "Extrude13" add sketch "Sketch10" along normal blind 30 contours L0 L1 L2 L6 L7 L8 L9
sketch "Sketch11" plane through (0, 5.5, 0) normal (0, -1, 0) x (1, 0, 0)
  line L0 (46, 36) -> (-16, 36)
  line L1 (-16, 36) -> (-16, 14)
  line L2 (-16, 14) -> (46, 14)
  line L3 (46, 14) -> (46, 36)
  line L4 (0, 31) -> (30, 31)
  line L5 (30, 31) -> (30, 21)
  line L6 (30, 21) -> (0, 21)
  line L7 (0, 21) -> (0, 31)
  line L8 (-16, 36) -> (46, 36)
  line L9 (46, 36) -> (46, 31)
  line L10 (46, 31) -> (-16, 31)
  line L11 (-16, 31) -> (-16, 36)
  constraint horizontal L8
  constraint vertical L9
  constraint horizontal L10
  constraint vertical L11
  constraint coincident L3 L9.end
  constraint coincident L0.end L1.start
extrude "Extrude14" add sketch "Sketch11" along normal blind 7 contours L0 L1 L3 L4 L8 L9 L10 L11
sketch "Sketch12" plane through (0, 0, 0) normal (1, 0, 0) x (0, 1, 0)
extrude "Extrude15" add 1 faces at (10, -1.5, 34.3333) along direction (0, -1, 0) blind 10
sketch "Sketch13" plane through (0, 0, 14) normal (0, 0, 1) x (-1, 0, 0)
  line L0 (-41, 71.5) -> (11, 71.5)
  line L1 (11, 71.5) -> (11, -0.5)
  line L2 (11, -0.5) -> (-41, -0.5)
  line L3 (-41, -0.5) -> (-41, 71.5)
  line L4 (-46, -5.5) -> (16, -5.5)
  line L5 (16, -5.5) -> (16, 76.5)
  line L6 (16, 76.5) -> (-46, 76.5)
  line L7 (-46, 76.5) -> (-46, -5.5)
  line L8 (-46, -5.5) -> (-41, -5.5)
  line L9 (-41, -5.5) -> (-41, 11.5)
  line L10 (-41, 11.5) -> (-46, 11.5)
  line L11 (-46, 11.5) -> (-46, -5.5)
  line L12 (-46, -5.5) -> (-30, -5.5)
  line L13 (-30, -5.5) -> (-30, -0.5)
  line L14 (-30, -0.5) -> (-46, -0.5)
  line L15 (-46, -0.5) -> (-46, -5.5)
  dimension "d138" = 17
  dimension "d139" = 16
  dimension "d140" = 5
  constraint horizontal L8
  constraint vertical L9
  constraint horizontal L10
  constraint vertical L11
  constraint coincident L4.start L7.end
  constraint horizontal L12
  constraint vertical L13
  constraint horizontal L14
  constraint vertical L15
  measures "d138" distance of L4.start L10.end
  measures "d139" distance of L4.start L12.end
  measures "d140" distance of L4.start L14.end
extrude "Extrude16" add sketch "Sketch13" along normal blind 17 contours L3 L7 L9 L10 L11 L14 | L2 L4 L9 L12 L13 L14 | L4 L7 L8 L9 L11 L12 L14 L15
sketch "Sketch14" plane through (0, 0, 14) normal (0, 0, 1) x (-1, 0, 0)
  line L0 (-30, -0.5) -> (-30, -5.5)
  line L1 (-30, -5.5) -> (16, -5.5)
  line L2 (16, -5.5) -> (16, 76.5)
  line L3 (16, 76.5) -> (-46, 76.5)
  line L4 (-46, 76.5) -> (-46, 11.5)
  line L5 (-46, 11.5) -> (-41, 11.5)
  line L6 (-41, 11.5) -> (-41, 71.5)
  line L7 (-41, 71.5) -> (11, 71.5)
  line L8 (11, 71.5) -> (11, -0.5)
  line L9 (11, -0.5) -> (-30, -0.5)
  line L10 (16, -5.5) -> (11, -5.5)
  line L11 (11, -5.5) -> (11, 11.5)
  line L12 (11, 11.5) -> (16, 11.5)
  line L13 (16, 11.5) -> (16, -5.5)
  line L14 (16, -5.5) -> (0, -5.5)
  line L15 (0, -5.5) -> (0, -0.5)
  line L16 (0, -0.5) -> (16, -0.5)
  line L17 (16, -0.5) -> (16, -5.5)
  dimension "d143" = 17
  constraint horizontal L10
  constraint vertical L11
  constraint horizontal L12
  constraint vertical L13
  constraint coincident L1.end L2.start
  constraint horizontal L14
  constraint vertical L15
  constraint horizontal L16
  constraint vertical L17
  constraint coincident L9 L15.end
  measures "d143" distance of L1.end L12.end
extrude "Extrude17" add sketch "Sketch14" along normal blind 17 contours L1 L9 L11 L14 L15 L16 | L1 L2 L10 L11 L13 L14 L16 L17 | L2 L8 L11 L12 L13 L16
extrude "Extrude18" cut 1 faces at (20, 6.5, 21) along direction (0, 0, -1) blind 7
sketch "Sketch15" plane through (0, 0, 36) normal (0, 0, 1) x (-1, 0, 0)
  line L0 (-46, -18.5) -> (16, -18.5)
  line L1 (16, -18.5) -> (16, 11.5)
  line L2 (16, 11.5) -> (-46, 11.5)
  line L3 (-46, 11.5) -> (-46, -18.5)
  line L4 (-15, -18.5) -> (-15, 11.5) construction
  line L5 (-15, -18.5) -> (-15, -16.5) construction
  line L6 (-15, -16.5) -> (-26.75, -16.5) construction
  line L7 (-26.75, -16.5) -> (-3.25, -16.5)
  line L8 (-3.25, -16.5) -> (-3.25, 10.5)
  line L9 (-3.25, 10.5) -> (-26.75, 10.5)
  line L10 (-26.75, 10.5) -> (-26.75, -16.5)
  line L11 (-26.75, 10.5) -> (-24.75, 10.5) construction
  line L12 (-24.75, 10.5) -> (-24.75, 8.5) construction
  line L13 (-24.75, 8.5) -> (-26.75, 8.5) construction
  line L14 (-26.75, 8.5) -> (-26.75, 10.5) construction
  line L15 (-24.75, 8.5) -> (-5.25, 8.5)
  line L16 (-5.25, 8.5) -> (-5.25, -15)
  line L17 (-5.25, -15) -> (-24.75, -15)
  line L18 (-24.75, -15) -> (-24.75, 8.5)
  dimension "d148" = 2
  dimension "d149" = 11.75
  dimension "d150" = 23.5
  dimension "d151" = 27
  dimension "d152" = 2
  dimension "d153" = 2
  dimension "d154" = 19.5
  constraint midpoint L0 L4.start
  constraint midpoint L2 L4.end
  constraint perpendicular L0 L5
  constraint perpendicular L5 L6
  constraint horizontal L7
  constraint vertical L8
  constraint horizontal L9
  constraint vertical L10
  constraint horizontal L11
  constraint vertical L12
  constraint horizontal L13
  constraint vertical L14
  constraint horizontal L15
  constraint vertical L16
  constraint horizontal L17
  constraint vertical L18
  measures "d148" distance of L4.start L5.end
  measures "d149" distance of L5.end L6.end
  measures "d150" distance of L6.end L7.end
  measures "d151" distance of L6.end L9.end
  measures "d152" distance of L9.end L11.end
  measures "d153" distance of L9.end L13.end
  measures "d154" distance of L12.end L15.end
extrude "Extrude19" add sketch "Sketch15" along normal blind 2 contours L7 L8 L9 L10
sketch "Sketch16" plane through (0, 0, 14) normal (0, 0, 1) x (-1, 0, 0)
  line L0 (11, 11.5) -> (16, 11.5)
  line L1 (16, 11.5) -> (16, 76.5)
  line L2 (16, 76.5) -> (-46, 76.5)
  line L3 (-46, 76.5) -> (-46, 11.5)
  line L4 (-46, 11.5) -> (-41, 11.5)
  line L5 (-41, 11.5) -> (-41, 71.5)
  line L6 (-41, 71.5) -> (11, 71.5)
  line L7 (11, 71.5) -> (11, 11.5)
  line L8 (-46, 76.5) -> (-31, 76.5) construction
  line L9 (-46, 76.5) -> (-46, 61.5) construction
  line L10 (16, 76.5) -> (1, 76.5) construction
  line L11 (16, 76.5) -> (16, 61.5) construction
  line L12 (-46, 61.5) -> (-41, 61.5)
  line L13 (-41, 61.5) -> (-41, 11.5)
  line L14 (-41, 11.5) -> (-46, 11.5)
  line L15 (-46, 11.5) -> (-46, 61.5)
  line L16 (-31, 76.5) -> (1, 76.5)
  line L17 (1, 76.5) -> (1, 71.5)
  line L18 (1, 71.5) -> (-31, 71.5)
  line L19 (-31, 71.5) -> (-31, 76.5)
  line L20 (16, 61.5) -> (11, 61.5)
  line L21 (11, 61.5) -> (11, 11.5)
  line L22 (11, 11.5) -> (16, 11.5)
  line L23 (16, 11.5) -> (16, 61.5)
  dimension "d157" = 15
  dimension "d158" = 15
  dimension "d159" = 15
  dimension "d160" = 15
  dimension "d161" = 32
  constraint coincident L2.end L3.start
  constraint perpendicular L3 L8
  constraint perpendicular L2 L9
  constraint coincident L1.end L2.start
  constraint perpendicular L1 L10
  constraint perpendicular L2 L11
  constraint horizontal L12
  constraint vertical L13
  constraint horizontal L14
  constraint vertical L15
  constraint coincident L4.end L5.start
  constraint horizontal L16
  constraint vertical L17
  constraint horizontal L18
  constraint vertical L19
  constraint horizontal L20
  constraint vertical L21
  constraint horizontal L22
  constraint vertical L23
  constraint coincident L0.start L7.end
  measures "d157" distance of L2.end L8.end
  measures "d158" distance of L2.end L9.end
  measures "d159" distance of L1.end L10.end
  measures "d160" distance of L1.end L11.end
  measures "d161" distance of L8.end L10.end
extrude "Extrude20" cut sketch "Sketch16" against normal blind 5 contours L0 L1 L7 L20 L21 L22 L23 | L2 L6 L16 L17 L18 L19 | L3 L4 L5 L12 L13 L14 L15
sketch "Sketch17" plane through (0, 0, 9) normal (0, 0, 1) x (-1, 0, 0)
  line L0 (-36, 4.5) -> (-36, 66.5)
  line L1 (-36, 66.5) -> (6, 66.5)
  line L2 (6, 66.5) -> (6, 4.5)
  line L3 (6, 4.5) -> (-36, 4.5)
  line L4 (-41, 71.5) -> (-41, 61.5)
  line L5 (-41, 61.5) -> (-46, 61.5)
  line L6 (-46, 61.5) -> (-46, 11.5)
  line L7 (-46, 11.5) -> (-41, 11.5)
  line L8 (-41, 11.5) -> (-41, -0.5)
  line L9 (-41, -0.5) -> (11, -0.5)
  line L10 (11, -0.5) -> (11, 11.5)
  line L11 (11, 11.5) -> (16, 11.5)
  line L12 (16, 11.5) -> (16, 61.5)
  line L13 (16, 61.5) -> (11, 61.5)
  line L14 (11, 61.5) -> (11, 71.5)
  line L15 (11, 71.5) -> (1, 71.5)
  line L16 (1, 71.5) -> (1, 76.5)
  line L17 (1, 76.5) -> (-31, 76.5)
  line L18 (-31, 76.5) -> (-31, 71.5)
  line L19 (-31, 71.5) -> (-41, 71.5)
  line L20 (11, 61.5) -> (16, 61.5)
  line L21 (16, 61.5) -> (16, 11.5)
  line L22 (16, 11.5) -> (11, 11.5)
  line L23 (11, 11.5) -> (11, 61.5)
  line L24 (-41, 61.5) -> (-46, 61.5)
  line L25 (-46, 61.5) -> (-46, 11.5)
  line L26 (-46, 11.5) -> (-41, 11.5)
  line L27 (-41, 11.5) -> (-41, 61.5)
  line L28 (1, 76.5) -> (-31, 76.5)
  line L29 (-31, 76.5) -> (-31, 71.5)
  line L30 (-31, 71.5) -> (1, 71.5)
  line L31 (1, 71.5) -> (1, 76.5)
  line L32 (-31, 71.5) -> (-41, 71.5)
  line L33 (-41, 71.5) -> (-41, 66.5)
  line L34 (-41, 66.5) -> (-31, 66.5)
  line L35 (-31, 66.5) -> (-31, 71.5)
  line L36 (-41, 61.5) -> (-36, 61.5)
  line L37 (-36, 61.5) -> (-36, 66)
  line L38 (-36, 66) -> (-41, 66)
  line L39 (-41, 66) -> (-41, 61.5)
  line L40 (11, 61.5) -> (6, 61.5)
  line L41 (6, 61.5) -> (6, 71.5)
  line L42 (6, 71.5) -> (11, 71.5)
  line L43 (11, 71.5) -> (11, 61.5)
  line L44 (1, 71.5) -> (6, 71.5)
  line L45 (6, 71.5) -> (6, 66.5)
  line L46 (6, 66.5) -> (1, 66.5)
  line L47 (1, 66.5) -> (1, 71.5)
  line L48 (-36, 66.5) -> (-41, 66.5)
  line L49 (-41, 66.5) -> (-41, 61.5)
  line L50 (-41, 61.5) -> (-36, 61.5)
  line L51 (-36, 61.5) -> (-36, 66.5)
  constraint horizontal L20
  constraint vertical L21
  constraint horizontal L22
  constraint vertical L23
  constraint coincident L11.end L12.start
  constraint coincident L13.end L14.start
  constraint horizontal L24
  constraint vertical L25
  constraint horizontal L26
  constraint vertical L27
  constraint coincident L6.end L7.start
  constraint coincident L4.end L5.start
  constraint horizontal L28
  constraint vertical L29
  constraint horizontal L30
  constraint vertical L31
  constraint coincident L18.end L19.start
  constraint coincident L16.end L17.start
  constraint horizontal L32
  constraint vertical L33
  constraint horizontal L34
  constraint vertical L35
  constraint midpoint L4 L33.end
  constraint horizontal L36
  constraint vertical L37
  constraint horizontal L38
  constraint vertical L39
  constraint coincident L0 L37.end
  constraint horizontal L40
  constraint vertical L41
  constraint horizontal L42
  constraint vertical L43
  constraint midpoint L15 L41.end
  constraint horizontal L44
  constraint vertical L45
  constraint horizontal L46
  constraint vertical L47
  constraint coincident L1.end L2.start
  constraint horizontal L48
  constraint vertical L49
  constraint horizontal L50
  constraint vertical L51
  constraint coincident L0.end L1.start
extrude "Extrude21" cut sketch "Sketch17" against normal blind 3 contours L0 L4 L36 L37 L38 L39 L49 L50 L51 | L5 L6 L7 L24 L25 L26 L27 | L2 L14 L15 L40 L41 L42 L43 L45 | L1 L4 L19 L32 L33 L34 L35 L48 | L1 L15 L41 L44 L45 L46 L47 | L11 L12 L13 L20 L21 L22 L23 | L16 L17 L18 L28 L29 L30 L31